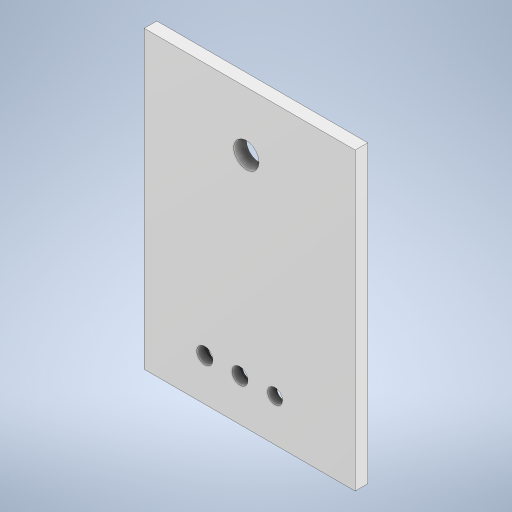
# Autodesk Inventor part: main base new edited new
Saved by Autodesk Inventor 2023 (Build 270158000, 158)
## iProperties
Created: 2022-06-23
Part Number: main base new edited new
Material: PVC, Unplasticized
Document SubType Name: Modeling
Designer: Anushree
Density: 1.29 g/cm^3
Appearance: Smooth - White
Author: Anushree
Autodesk Inventor part; units mm, degrees
ref_plane "YZ Plane" through (0, 0, 0) normal (1, 0, 0) x (0, 1, 0)
ref_plane "XZ Plane" through (0, 0, 0) normal (0, 1, 0) x (-1, 0, 0)
ref_plane "XY Plane" through (0, 0, 0) normal (0, 0, 1) x (1, 0, 0)
sketch "Sketch1" plane through (0, 0, 0) normal (0, 0, 1) x (1, 0, 0)
  line L0 (-9.3024, 8.297) -> (240.6976, 8.297)
  line L1 (240.6976, 8.297) -> (240.6976, -341.703)
  line L2 (240.6976, -341.703) -> (-9.3024, -341.703)
  line L3 (-9.3024, -341.703) -> (-9.3024, 8.297)
  point P0 (0, 0)
  dimension "d0" = 250
  dimension "d1" = 350
  constraints: 8 end point, 2 parallel, 1 horizontal, 1 perpendicular
  measures "d0" distance of L1.end L2.end
  measures "d1" distance of L0.end L1.end
extrude "Extrusion1" add sketch "Sketch1" along normal blind 15
sketch "Sketch2" plane through (0, 0, 15) normal (0, 0, 1) x (1, 0, 0)
  circle A0 centre (104.1886, -291.703) radius 9.5908
  circle A1 centre (62.5936, -291.703) radius 9.5908
  line L0 (240.6976, 8.297) -> (-9.3024, 8.297) projected
  line L1 (-9.3024, -341.703) -> (240.6976, -341.703) projected
  line L2 (240.6976, -341.703) -> (240.6976, 8.297) projected
  circle A2 centre (145.7836, -291.703) radius 8.9222
  line L3 (-9.3024, 8.297) -> (-9.3024, -341.703) projected
  point P0 (0, 0)
  point P1 (115.6976, -341.703)
  constraints: 3 centre point, 1 midpoint
extrude "Extrusion2" cut sketch "Sketch2" against normal blind 10 contours A0 | A1 | A2
sketch "Sketch3" plane through (62.5936, -291.703, 5) normal (0, 0, 1) x (1, 0, 0)
  point P0 (-62.5936, 291.703)
  point P1 (-0.6647, -4.2616)
hole "Hole1" at (61.9289, -295.9646, 5) direction (0, 0, -1) diameter 20 end through all
sketch "Sketch4" plane through (104.1886, -291.703, 5) normal (0, 0, 1) x (1, 0, 0)
  point P0 (-104.1886, 291.703)
  point P1 (-2.459, -3.2991)
hole "Hole2" at (101.7296, -295.0021, 5) direction (0, 0, -1) diameter 20 end through all
sketch "Sketch5" plane through (145.7836, -291.703, 5) normal (0, 0, 1) x (1, 0, 0)
  point P0 (-145.7836, 291.703)
  point P1 (-3.1106, -5.2364)
hole "Hole3" at (142.673, -296.9394, 5) direction (0, 0, -1) diameter 20 end through all
sketch "Sketch6" plane through (0, 0, 15) normal (0, 0, 1) x (1, 0, 0)
  circle A0 centre (111.8077, -61.2607) radius 10
  point P0 (0, 0)
  dimension "d41" = 20
  constraints: 1 centre point
  measures "d41" diameter of A0
hole "Hole4" at (111.8077, -61.2607, 15) direction (0, 0, -1) diameter 20 end through all
sketch "Sketch7" plane through (0, 0, 15) normal (0, 0, 1) x (1, 0, 0)
  circle A0 centre (111.8077, -61.2607) radius 10 projected
  circle A1 centre (111.8077, -61.2607) radius 15
  point P0 (0, 0)
  dimension "d49" = 30
  constraints: 1 centre point, 1 coincident
  measures "d49" diameter of A1
hole "Hole5" at (111.8077, -61.2607, 15) direction (0, 0, -1) diameter 30 end through all
body "Solid1"
